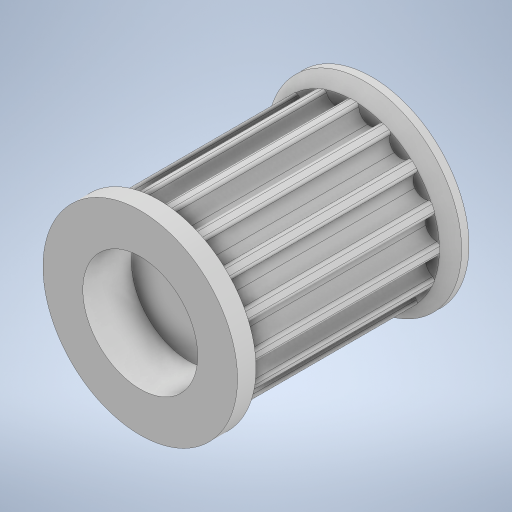
# Autodesk Inventor part: y_idler_teeth
Saved by Autodesk Inventor 2023 (Build 270158030, 158C)
## iProperties
Created: 2022-06-27
Part Number: y_idler_teeth
Material: 一般
Document SubType Name: Modeling
Designer: user
Density: 1 g/cm^3
Appearance: 預設
Author: user
## iProperties of the stored document y_idler_teeth_6mm_3D 列印.ipt
Created: 2022-06-29
Part Number: y_idler_teeth_6mm_3D 列印
Material: 一般
Document SubType Name: Modeling
Designer: user
Density: 1 g/cm^3
Appearance: 預設
Author: user
Autodesk Inventor part; units mm, degrees
ref_plane "YZ Plane" through (0, 0, 0) normal (1, 0, 0) x (0, 1, 0)
ref_plane "XZ Plane" through (0, 0, 0) normal (0, 1, 0) x (-1, 0, 0)
ref_plane "XY Plane" through (0, 0, 0) normal (0, 0, 1) x (1, 0, 0)
sketch "草圖1" plane through (0, 0, 0) normal (0, 0, 1) x (1, 0, 0)
  circle A0 centre (0, 0) radius 4
  arc A1 (0.305, 4.510097) -> (0.786957, 3.921823) centre (0.905, 4.510097) ccw
  arc A2 (-0.786957, 3.921823) -> (-0.305, 4.510097) centre (-0.905, 4.510097) ccw
  line L0 (0, -7) -> (0, 7)
  line L1 (-0.305, 4.510097) -> (0.305, 4.510097)
  line L2 (0.305, 4.510097) -> (0.305, 4.512097)
  line L3 (0.155, 4.662097) -> (-0.155, 4.662097)
  line L4 (-0.305, 4.512097) -> (-0.305, 4.510097)
  arc A3 (-0.155, 4.662097) -> (-0.305, 4.512097) centre (-0.155, 4.512097) ccw
  arc A4 (0.305, 4.512097) -> (0.155, 4.662097) centre (0.155, 4.512097) ccw
  circle A5 centre (0, 0) radius 3.1
  arc A6 (-2.22787, 3.322137) -> (-2.007723, 4.050068) centre (-2.56205, 3.820458) ccw
  line L5 (-1.640906, 4.366532) -> (-1.927309, 4.2479)
  arc A7 (-1.927309, 4.2479) -> (-2.008488, 4.051916) centre (-1.869906, 4.109318) ccw
  arc A8 (-1.444922, 4.285353) -> (-1.640906, 4.366532) centre (-1.583503, 4.22795) ccw
  arc A9 (-1.444156, 4.283505) -> (-0.773764, 3.924448) centre (-0.889828, 4.513115) ccw
  arc A10 (-3.32961, 2.216686) -> (-3.404788, 2.973453) centre (-3.829052, 2.549189) ccw
  line L6 (-3.186999, 3.406202) -> (-3.406202, 3.186999)
  arc A11 (-3.406202, 3.186999) -> (-3.406202, 2.974867) centre (-3.300136, 3.080933) ccw
  arc A12 (-2.974867, 3.406202) -> (-3.186999, 3.406202) centre (-3.080933, 3.300136) ccw
  arc A13 (-2.973453, 3.404788) -> (-2.216686, 3.32961) centre (-2.549189, 3.829052) ccw
  arc A14 (-3.924448, 0.773764) -> (-4.283505, 1.444156) centre (-4.513115, 0.889828) ccw
  line L7 (-4.2479, 1.927309) -> (-4.366532, 1.640906)
  arc A15 (-4.366532, 1.640906) -> (-4.285353, 1.444922) centre (-4.22795, 1.583503) ccw
  arc A16 (-4.051916, 2.008488) -> (-4.2479, 1.927309) centre (-4.109318, 1.869906) ccw
  arc A17 (-4.050068, 2.007723) -> (-3.322137, 2.22787) centre (-3.820458, 2.56205) ccw
  arc A18 (-3.921823, -0.786957) -> (-4.510097, -0.305) centre (-4.510097, -0.905) ccw
  line L8 (-4.662097, 0.155) -> (-4.662097, -0.155)
  arc A19 (-4.662097, -0.155) -> (-4.512097, -0.305) centre (-4.512097, -0.155) ccw
  arc A20 (-4.512097, 0.305) -> (-4.662097, 0.155) centre (-4.512097, 0.155) ccw
  arc A21 (-4.510097, 0.305) -> (-3.921823, 0.786957) centre (-4.510097, 0.905) ccw
  arc A22 (-3.322137, -2.22787) -> (-4.050068, -2.007723) centre (-3.820458, -2.56205) ccw
  line L9 (-4.366532, -1.640906) -> (-4.2479, -1.927309)
  arc A23 (-4.2479, -1.927309) -> (-4.051916, -2.008488) centre (-4.109318, -1.869906) ccw
  arc A24 (-4.285353, -1.444922) -> (-4.366532, -1.640906) centre (-4.22795, -1.583503) ccw
  arc A25 (-4.283505, -1.444156) -> (-3.924448, -0.773764) centre (-4.513115, -0.889828) ccw
  arc A26 (-2.216686, -3.32961) -> (-2.973453, -3.404788) centre (-2.549189, -3.829052) ccw
  line L10 (-3.406202, -3.186999) -> (-3.186999, -3.406202)
  arc A27 (-3.186999, -3.406202) -> (-2.974867, -3.406202) centre (-3.080933, -3.300136) ccw
  arc A28 (-3.406202, -2.974867) -> (-3.406202, -3.186999) centre (-3.300136, -3.080933) ccw
  arc A29 (-3.404788, -2.973453) -> (-3.32961, -2.216686) centre (-3.829052, -2.549189) ccw
  arc A30 (-0.773764, -3.924448) -> (-1.444156, -4.283505) centre (-0.889828, -4.513115) ccw
  line L11 (-1.927309, -4.2479) -> (-1.640906, -4.366532)
  arc A31 (-1.640906, -4.366532) -> (-1.444922, -4.285353) centre (-1.583503, -4.22795) ccw
  arc A32 (-2.008488, -4.051916) -> (-1.927309, -4.2479) centre (-1.869906, -4.109318) ccw
  arc A33 (-2.007723, -4.050068) -> (-2.22787, -3.322137) centre (-2.56205, -3.820458) ccw
  arc A34 (0.786957, -3.921823) -> (0.305, -4.510097) centre (0.905, -4.510097) ccw
  line L12 (-0.155, -4.662097) -> (0.155, -4.662097)
  arc A35 (0.155, -4.662097) -> (0.305, -4.512097) centre (0.155, -4.512097) ccw
  arc A36 (-0.305, -4.512097) -> (-0.155, -4.662097) centre (-0.155, -4.512097) ccw
  arc A37 (-0.305, -4.510097) -> (-0.786957, -3.921823) centre (-0.905, -4.510097) ccw
  arc A38 (2.22787, -3.322137) -> (2.007723, -4.050068) centre (2.56205, -3.820458) ccw
  line L13 (1.640906, -4.366532) -> (1.927309, -4.2479)
  arc A39 (1.927309, -4.2479) -> (2.008488, -4.051916) centre (1.869906, -4.109318) ccw
  arc A40 (1.444922, -4.285353) -> (1.640906, -4.366532) centre (1.583503, -4.22795) ccw
  arc A41 (1.444156, -4.283505) -> (0.773764, -3.924448) centre (0.889828, -4.513115) ccw
  arc A42 (3.32961, -2.216686) -> (3.404788, -2.973453) centre (3.829052, -2.549189) ccw
  line L14 (3.186999, -3.406202) -> (3.406202, -3.186999)
  arc A43 (3.406202, -3.186999) -> (3.406202, -2.974867) centre (3.300136, -3.080933) ccw
  arc A44 (2.974867, -3.406202) -> (3.186999, -3.406202) centre (3.080933, -3.300136) ccw
  arc A45 (2.973453, -3.404788) -> (2.216686, -3.32961) centre (2.549189, -3.829052) ccw
  arc A46 (3.924448, -0.773764) -> (4.283505, -1.444156) centre (4.513115, -0.889828) ccw
  line L15 (4.2479, -1.927309) -> (4.366532, -1.640906)
  arc A47 (4.366532, -1.640906) -> (4.285353, -1.444922) centre (4.22795, -1.583503) ccw
  arc A48 (4.051916, -2.008488) -> (4.2479, -1.927309) centre (4.109318, -1.869906) ccw
  arc A49 (4.050068, -2.007723) -> (3.322137, -2.22787) centre (3.820458, -2.56205) ccw
  arc A50 (3.921823, 0.786957) -> (4.510097, 0.305) centre (4.510097, 0.905) ccw
  line L16 (4.662097, -0.155) -> (4.662097, 0.155)
  arc A51 (4.662097, 0.155) -> (4.512097, 0.305) centre (4.512097, 0.155) ccw
  arc A52 (4.512097, -0.305) -> (4.662097, -0.155) centre (4.512097, -0.155) ccw
  arc A53 (4.510097, -0.305) -> (3.921823, -0.786957) centre (4.510097, -0.905) ccw
  arc A54 (3.322137, 2.22787) -> (4.050068, 2.007723) centre (3.820458, 2.56205) ccw
  line L17 (4.366532, 1.640906) -> (4.2479, 1.927309)
  arc A55 (4.2479, 1.927309) -> (4.051916, 2.008488) centre (4.109318, 1.869906) ccw
  arc A56 (4.285353, 1.444922) -> (4.366532, 1.640906) centre (4.22795, 1.583503) ccw
  arc A57 (4.283505, 1.444156) -> (3.924448, 0.773764) centre (4.513115, 0.889828) ccw
  arc A58 (2.216686, 3.32961) -> (2.973453, 3.404788) centre (2.549189, 3.829052) ccw
  line L18 (3.406202, 3.186999) -> (3.186999, 3.406202)
  arc A59 (3.186999, 3.406202) -> (2.974867, 3.406202) centre (3.080933, 3.300136) ccw
  arc A60 (3.406202, 2.974867) -> (3.406202, 3.186999) centre (3.300136, 3.080933) ccw
  arc A61 (3.404788, 2.973453) -> (3.32961, 2.216686) centre (3.829052, 2.549189) ccw
  arc A62 (0.773764, 3.924448) -> (1.444156, 4.283505) centre (0.889828, 4.513115) ccw
  line L19 (1.927309, 4.2479) -> (1.640906, 4.366532)
  arc A63 (1.640906, 4.366532) -> (1.444922, 4.285353) centre (1.583503, 4.22795) ccw
  arc A64 (2.008488, 4.051916) -> (1.927309, 4.2479) centre (1.869906, 4.109318) ccw
  arc A65 (2.007723, 4.050068) -> (2.22787, 3.322137) centre (2.56205, 3.820458) ccw
  circle A66 centre (0, 0) radius 5
  line L20 (-1.444925, 4.28536) -> (-1.444156, 4.283505)
  line L21 (-2.008488, 4.051916) -> (-2.007723, 4.050068)
  line L22 (-3.406202, 2.974867) -> (-3.404788, 2.973453)
  line L23 (-2.974873, 3.406208) -> (-2.973453, 3.404788)
  line L24 (-4.285353, 1.444922) -> (-4.283505, 1.444156)
  line L25 (-4.051923, 2.008491) -> (-4.050068, 2.007723)
  line L26 (-4.512097, -0.305) -> (-4.510097, -0.305)
  line L27 (-4.512105, 0.305) -> (-4.510097, 0.305)
  line L28 (-4.051916, -2.008488) -> (-4.050068, -2.007723)
  line L29 (-4.28536, -1.444925) -> (-4.283505, -1.444156)
  line L30 (-2.974867, -3.406202) -> (-2.973453, -3.404788)
  line L31 (-3.406208, -2.974873) -> (-3.404788, -2.973453)
  line L32 (-1.444922, -4.285353) -> (-1.444156, -4.283505)
  line L33 (-2.008491, -4.051923) -> (-2.007723, -4.050068)
  line L34 (0.305, -4.512097) -> (0.305, -4.510097)
  line L35 (-0.305, -4.512105) -> (-0.305, -4.510097)
  line L36 (2.008488, -4.051916) -> (2.007723, -4.050068)
  line L37 (1.444925, -4.28536) -> (1.444156, -4.283505)
  line L38 (3.406202, -2.974867) -> (3.404788, -2.973453)
  line L39 (2.974873, -3.406208) -> (2.973453, -3.404788)
  line L40 (4.285353, -1.444922) -> (4.283505, -1.444156)
  line L41 (4.051923, -2.008491) -> (4.050068, -2.007723)
  line L42 (4.512097, 0.305) -> (4.510097, 0.305)
  line L43 (4.512105, -0.305) -> (4.510097, -0.305)
  line L44 (4.051916, 2.008488) -> (4.050068, 2.007723)
  line L45 (4.28536, 1.444925) -> (4.283505, 1.444156)
  line L46 (2.974867, 3.406202) -> (2.973453, 3.404788)
  line L47 (3.406208, 2.974873) -> (3.404788, 2.973453)
  line L48 (1.444922, 4.285353) -> (1.444156, 4.283505)
  line L49 (2.008491, 4.051923) -> (2.007723, 4.050068)
  line L50 (-0.305, 4.512097) -> (-0.305, 4.510097)
  line L51 (0.305, 4.512105) -> (0.305, 4.510097)
  circle A67 centre (0, 0) radius 2
  point P0 (-0.78037, 3.923184)
  point P1 (-2.222305, 3.325914)
  point P2 (-3.404788, 2.973453)
  point P3 (-3.325914, 2.222305)
  point P4 (-3.923184, 0.78037)
  point P5 (-4.512097, 0.305)
  point P6 (-4.512097, -0.305)
  point P7 (-4.510097, -0.305)
  point P8 (-3.923184, -0.78037)
  point P9 (-4.283505, -1.444156)
  point P10 (-3.325914, -2.222305)
  point P11 (-2.222305, -3.325914)
  point P12 (-0.78037, -3.923184)
  point P13 (-0.305, -4.512097)
  point P14 (0.305, -4.512097)
  point P15 (0.78037, -3.923184)
  point P16 (2.222305, -3.325914)
  point P17 (3.325914, -2.222305)
  point P18 (4.283505, -1.444156)
  point P19 (3.923184, -0.78037)
  point P20 (4.512097, -0.305)
  point P21 (4.512097, 0.305)
  point P22 (3.923184, 0.78037)
  point P23 (4.283505, 1.444156)
  point P24 (4.051916, 2.008488)
  point P25 (3.325914, 2.222305)
  point P26 (2.973453, 3.404788)
  point P27 (2.222305, 3.325914)
  point P28 (1.444922, 4.285353)
  point P29 (0.78037, 3.923184)
  dimension "d0" = 8
  dimension "d1" = 1.2
  dimension "d2" = 0.61
  dimension "d3" = 0.15
  dimension "d4" = 0.152
  dimension "d5" = 6.2
  dimension "d8" = 360
  dimension "d10" = 10
  dimension "d13" = 360
  dimension "d20" = 4
  constraints: 130 point on circle, 102 end point, 68 centre point, 8 tangent, 4 coincident, 3 parallel, 1 equal radius, 1 horizontal, 1 perpendicular, 1 symmetric about line, 370 other
  measures "d0" diameter of A0
  measures "d1" diameter of A2
  measures "d2" distance of L1.start L1.end
  measures "d3" radius of A3
  measures "d4" distance between parallel lines of L1 L3
  measures "d5" diameter of A5
  measures "d10" diameter of A66
  measures "d20" diameter of A67
extrude "擠出1" add sketch "草圖1" along normal mid plane 10.5 contours A0 L0 A5 | A0 A50 A51 L16 A52 A53 | A0 A54 A55 L17 A56 A57 | A46 A47 L15 A48 A49 A0 | A0 A58 A59 L18 A60 A61 | A42 A43 L14 A44 A45 A0 | A0 A62 A63 L19 A64 A65 | A38 A39 L13 A40 A41 A0 | A0 L0 L1 A1 | A34 A35 L12 L0 A0 | L0 A5 A0 | A0 A2 L1 L0 | L1 L0 L3 A4 | L0 L12 A36 A37 A0 | L1 A3 L3 L0 | A0 A6 A7 L5 A8 A9 | A30 A31 L11 A32 A33 A0 | A0 A10 A11 L6 A12 A13 | A26 A27 L10 A28 A29 A0 | A0 A14 A15 L7 A16 A17 | A22 A23 L9 A24 A25 A0 | A0 A18 A19 L8 A20 A21
sketch "草圖2" plane through (0, 0, 5.25) normal (0, 0, 1) x (1, 0, 0)
  arc A0 (-1.444922, 4.285353) -> (-0.78037, 3.923184) centre (-0.889827, 4.513123) ccw
  arc A1 (-1.444922, 4.285353) -> (-1.640906, 4.366532) centre (-1.583503, 4.22795) ccw
  line L0 (-1.640906, 4.366532) -> (-1.927309, 4.2479)
  arc A2 (-1.927309, 4.2479) -> (-2.008488, 4.051916) centre (-1.869906, 4.109318) ccw
  arc A3 (-2.222305, 3.325914) -> (-2.008488, 4.051916) centre (-2.562057, 3.820462) ccw
  arc A4 (-2.974867, 3.406202) -> (-2.222305, 3.325914) centre (-2.54919, 3.829059) ccw
  arc A5 (-2.974867, 3.406202) -> (-3.186999, 3.406202) centre (-3.080933, 3.300136) ccw
  line L1 (-3.186999, 3.406202) -> (-3.406202, 3.186999)
  arc A6 (-3.406202, 3.186999) -> (-3.406202, 2.974867) centre (-3.300136, 3.080933) ccw
  arc A7 (-3.325914, 2.222305) -> (-3.406202, 2.974867) centre (-3.829059, 2.54919) ccw
  arc A8 (-4.051916, 2.008488) -> (-3.325914, 2.222305) centre (-3.820462, 2.562057) ccw
  arc A9 (-4.051916, 2.008488) -> (-4.2479, 1.927309) centre (-4.109318, 1.869906) ccw
  line L2 (-4.2479, 1.927309) -> (-4.366532, 1.640906)
  arc A10 (-4.366532, 1.640906) -> (-4.285353, 1.444922) centre (-4.22795, 1.583503) ccw
  arc A11 (-3.923184, 0.78037) -> (-4.285353, 1.444922) centre (-4.513123, 0.889827) ccw
  arc A12 (-4.512097, 0.305) -> (-3.923184, 0.78037) centre (-4.510104, 0.905004) ccw
  arc A13 (-4.512097, 0.305) -> (-4.662097, 0.155) centre (-4.512097, 0.155) ccw
  line L3 (-4.662097, 0.155) -> (-4.662097, -0.155)
  arc A14 (-4.662097, -0.155) -> (-4.512097, -0.305) centre (-4.512097, -0.155) ccw
  arc A15 (-3.923184, -0.78037) -> (-4.512097, -0.305) centre (-4.510104, -0.905004) ccw
  arc A16 (-4.285353, -1.444922) -> (-3.923184, -0.78037) centre (-4.513123, -0.889827) ccw
  arc A17 (-4.285353, -1.444922) -> (-4.366532, -1.640906) centre (-4.22795, -1.583503) ccw
  line L4 (-4.366532, -1.640906) -> (-4.2479, -1.927309)
  arc A18 (-4.2479, -1.927309) -> (-4.051916, -2.008488) centre (-4.109318, -1.869906) ccw
  arc A19 (-3.325914, -2.222305) -> (-4.051916, -2.008488) centre (-3.820462, -2.562057) ccw
  arc A20 (-3.406202, -2.974867) -> (-3.325914, -2.222305) centre (-3.829059, -2.54919) ccw
  arc A21 (-3.406202, -2.974867) -> (-3.406202, -3.186999) centre (-3.300136, -3.080933) ccw
  line L5 (-3.406202, -3.186999) -> (-3.186999, -3.406202)
  arc A22 (-3.186999, -3.406202) -> (-2.974867, -3.406202) centre (-3.080933, -3.300136) ccw
  arc A23 (-2.222305, -3.325914) -> (-2.974867, -3.406202) centre (-2.54919, -3.829059) ccw
  arc A24 (-2.008488, -4.051916) -> (-2.222305, -3.325914) centre (-2.562057, -3.820462) ccw
  arc A25 (-2.008488, -4.051916) -> (-1.927309, -4.2479) centre (-1.869906, -4.109318) ccw
  line L6 (-1.927309, -4.2479) -> (-1.640906, -4.366532)
  arc A26 (-1.640906, -4.366532) -> (-1.444922, -4.285353) centre (-1.583503, -4.22795) ccw
  arc A27 (-0.78037, -3.923184) -> (-1.444922, -4.285353) centre (-0.889827, -4.513123) ccw
  arc A28 (-0.305, -4.512097) -> (-0.78037, -3.923184) centre (-0.905004, -4.510104) ccw
  arc A29 (-0.305, -4.512097) -> (-0.155, -4.662097) centre (-0.155, -4.512097) ccw
  line L7 (-0.155, -4.662097) -> (0.155, -4.662097)
  arc A30 (0.155, -4.662097) -> (0.305, -4.512097) centre (0.155, -4.512097) ccw
  arc A31 (0.78037, -3.923184) -> (0.305, -4.512097) centre (0.905004, -4.510104) ccw
  arc A32 (1.444922, -4.285353) -> (0.78037, -3.923184) centre (0.889827, -4.513123) ccw
  arc A33 (1.444922, -4.285353) -> (1.640906, -4.366532) centre (1.583503, -4.22795) ccw
  line L8 (1.640906, -4.366532) -> (1.927309, -4.2479)
  arc A34 (1.927309, -4.2479) -> (2.008488, -4.051916) centre (1.869906, -4.109318) ccw
  arc A35 (2.222305, -3.325914) -> (2.008488, -4.051916) centre (2.562057, -3.820462) ccw
  arc A36 (2.974867, -3.406202) -> (2.222305, -3.325914) centre (2.54919, -3.829059) ccw
  arc A37 (2.974867, -3.406202) -> (3.186999, -3.406202) centre (3.080933, -3.300136) ccw
  line L9 (3.186999, -3.406202) -> (3.406202, -3.186999)
  arc A38 (3.406202, -3.186999) -> (3.406202, -2.974867) centre (3.300136, -3.080933) ccw
  arc A39 (3.325914, -2.222305) -> (3.406202, -2.974867) centre (3.829059, -2.54919) ccw
  arc A40 (4.051916, -2.008488) -> (3.325914, -2.222305) centre (3.820462, -2.562057) ccw
  arc A41 (4.051916, -2.008488) -> (4.2479, -1.927309) centre (4.109318, -1.869906) ccw
  line L10 (4.2479, -1.927309) -> (4.366532, -1.640906)
  arc A42 (4.366532, -1.640906) -> (4.285353, -1.444922) centre (4.22795, -1.583503) ccw
  arc A43 (3.923184, -0.78037) -> (4.285353, -1.444922) centre (4.513123, -0.889827) ccw
  arc A44 (4.512097, -0.305) -> (3.923184, -0.78037) centre (4.510104, -0.905004) ccw
  arc A45 (4.512097, -0.305) -> (4.662097, -0.155) centre (4.512097, -0.155) ccw
  line L11 (4.662097, -0.155) -> (4.662097, 0.155)
  arc A46 (4.662097, 0.155) -> (4.512097, 0.305) centre (4.512097, 0.155) ccw
  arc A47 (3.923184, 0.78037) -> (4.512097, 0.305) centre (4.510104, 0.905004) ccw
  arc A48 (4.285353, 1.444922) -> (3.923184, 0.78037) centre (4.513123, 0.889827) ccw
  arc A49 (4.285353, 1.444922) -> (4.366532, 1.640906) centre (4.22795, 1.583503) ccw
  line L12 (4.366532, 1.640906) -> (4.2479, 1.927309)
  arc A50 (4.2479, 1.927309) -> (4.051916, 2.008488) centre (4.109318, 1.869906) ccw
  arc A51 (3.325914, 2.222305) -> (4.051916, 2.008488) centre (3.820462, 2.562057) ccw
  arc A52 (3.406202, 2.974867) -> (3.325914, 2.222305) centre (3.829059, 2.54919) ccw
  arc A53 (3.406202, 2.974867) -> (3.406202, 3.186999) centre (3.300136, 3.080933) ccw
  line L13 (3.406202, 3.186999) -> (3.186999, 3.406202)
  arc A54 (3.186999, 3.406202) -> (2.974867, 3.406202) centre (3.080933, 3.300136) ccw
  arc A55 (2.222305, 3.325914) -> (2.974867, 3.406202) centre (2.54919, 3.829059) ccw
  arc A56 (2.008488, 4.051916) -> (2.222305, 3.325914) centre (2.562057, 3.820462) ccw
  arc A57 (2.008488, 4.051916) -> (1.927309, 4.2479) centre (1.869906, 4.109318) ccw
  line L14 (1.927309, 4.2479) -> (1.640906, 4.366532)
  arc A58 (1.640906, 4.366532) -> (1.444922, 4.285353) centre (1.583503, 4.22795) ccw
  arc A59 (0.78037, 3.923184) -> (1.444922, 4.285353) centre (0.889827, 4.513123) ccw
  arc A60 (0.305, 4.512097) -> (0.78037, 3.923184) centre (0.905004, 4.510104) ccw
  arc A61 (0.305, 4.512097) -> (0.155, 4.662097) centre (0.155, 4.512097) ccw
  line L15 (0.155, 4.662097) -> (-0.155, 4.662097)
  arc A62 (-0.155, 4.662097) -> (-0.305, 4.512097) centre (-0.155, 4.512097) ccw
  arc A63 (-0.78037, 3.923184) -> (-0.305, 4.512097) centre (-0.905004, 4.510104) ccw
  circle A64 centre (0, 0) radius 3.1
  circle A65 centre (0, 0) radius 5.25
  dimension "d17" = 10.5
  constraints: 1 centre point, 1 coincident
  measures "d17" diameter of A65
extrude "擠出2" add sketch "草圖2" along normal blind 1 contours A0 A63 A62 L15 A61 A60 A59 A58 L14 A57 A56 A55 A54 L13 A53 A52 A51 A50 L12 A49 A48 A47 A46 L11 A45 A44 A43 A42 L10 A41 A40 A39 A38 L9 A37 A36 A35 A34 L8 A33 A32 A31 A30 L7 A29 A28 A27 A26 L6 A25 A24 A23 A22 L5 A21 A20 A19 A18 L4 A17 A16 A15 A14 L3 A13 A12 A11 A10 L2 A9 A8 A7 A6 L1 A5 A4 A3 A2 L0 A1 | A65
mirror "鏡射1" about plane through (0, 0, 0) normal (0, 0, 1) of "擠出2"
extrude "擠出3" add sketch "草圖1" along normal mid plane 7.25 contours A5 L0 A67 | L0 A67 A5
sketch "草圖3" plane through (0, 0, 3.625) normal (0, 0, 1) x (1, 0, 0)
  circle A0 centre (0, 0) radius 2
  circle A1 centre (0, 0) radius 3.1
  arc A2 (-0.78037, 3.923184) -> (-0.305, 4.512097) centre (-0.905004, 4.510104) ccw
  arc A3 (-0.155, 4.662097) -> (-0.305, 4.512097) centre (-0.155, 4.512097) ccw
  line L0 (-0.155, 4.662097) -> (0.155, 4.662097)
  arc A4 (0.305, 4.512097) -> (0.155, 4.662097) centre (0.155, 4.512097) ccw
  arc A5 (0.305, 4.512097) -> (0.78037, 3.923184) centre (0.905004, 4.510104) ccw
  arc A6 (0.78037, 3.923184) -> (1.444922, 4.285353) centre (0.889827, 4.513123) ccw
  arc A7 (1.640906, 4.366532) -> (1.444922, 4.285353) centre (1.583503, 4.22795) ccw
  line L1 (1.640906, 4.366532) -> (1.927309, 4.2479)
  arc A8 (2.008488, 4.051916) -> (1.927309, 4.2479) centre (1.869906, 4.109318) ccw
  arc A9 (2.008488, 4.051916) -> (2.222305, 3.325914) centre (2.562057, 3.820462) ccw
  arc A10 (2.222305, 3.325914) -> (2.974867, 3.406202) centre (2.54919, 3.829059) ccw
  arc A11 (3.186999, 3.406202) -> (2.974867, 3.406202) centre (3.080933, 3.300136) ccw
  line L2 (3.186999, 3.406202) -> (3.406202, 3.186999)
  arc A12 (3.406202, 2.974867) -> (3.406202, 3.186999) centre (3.300136, 3.080933) ccw
  arc A13 (3.406202, 2.974867) -> (3.325914, 2.222305) centre (3.829059, 2.54919) ccw
  arc A14 (3.325914, 2.222305) -> (4.051916, 2.008488) centre (3.820462, 2.562057) ccw
  arc A15 (4.2479, 1.927309) -> (4.051916, 2.008488) centre (4.109318, 1.869906) ccw
  line L3 (4.2479, 1.927309) -> (4.366532, 1.640906)
  arc A16 (4.285353, 1.444922) -> (4.366532, 1.640906) centre (4.22795, 1.583503) ccw
  arc A17 (4.285353, 1.444922) -> (3.923184, 0.78037) centre (4.513123, 0.889827) ccw
  arc A18 (3.923184, 0.78037) -> (4.512097, 0.305) centre (4.510104, 0.905004) ccw
  arc A19 (4.662097, 0.155) -> (4.512097, 0.305) centre (4.512097, 0.155) ccw
  line L4 (4.662097, 0.155) -> (4.662097, -0.155)
  arc A20 (4.512097, -0.305) -> (4.662097, -0.155) centre (4.512097, -0.155) ccw
  arc A21 (4.512097, -0.305) -> (3.923184, -0.78037) centre (4.510104, -0.905004) ccw
  arc A22 (3.923184, -0.78037) -> (4.285353, -1.444922) centre (4.513123, -0.889827) ccw
  arc A23 (4.366532, -1.640906) -> (4.285353, -1.444922) centre (4.22795, -1.583503) ccw
  line L5 (4.366532, -1.640906) -> (4.2479, -1.927309)
  arc A24 (4.051916, -2.008488) -> (4.2479, -1.927309) centre (4.109318, -1.869906) ccw
  arc A25 (4.051916, -2.008488) -> (3.325914, -2.222305) centre (3.820462, -2.562057) ccw
  arc A26 (3.325914, -2.222305) -> (3.406202, -2.974867) centre (3.829059, -2.54919) ccw
  arc A27 (3.406202, -3.186999) -> (3.406202, -2.974867) centre (3.300136, -3.080933) ccw
  line L6 (3.406202, -3.186999) -> (3.186999, -3.406202)
  arc A28 (2.974867, -3.406202) -> (3.186999, -3.406202) centre (3.080933, -3.300136) ccw
  arc A29 (2.974867, -3.406202) -> (2.222305, -3.325914) centre (2.54919, -3.829059) ccw
  arc A30 (2.222305, -3.325914) -> (2.008488, -4.051916) centre (2.562057, -3.820462) ccw
  arc A31 (1.927309, -4.2479) -> (2.008488, -4.051916) centre (1.869906, -4.109318) ccw
  line L7 (1.927309, -4.2479) -> (1.640906, -4.366532)
  arc A32 (1.444922, -4.285353) -> (1.640906, -4.366532) centre (1.583503, -4.22795) ccw
  arc A33 (1.444922, -4.285353) -> (0.78037, -3.923184) centre (0.889827, -4.513123) ccw
  arc A34 (0.78037, -3.923184) -> (0.305, -4.512097) centre (0.905004, -4.510104) ccw
  arc A35 (0.155, -4.662097) -> (0.305, -4.512097) centre (0.155, -4.512097) ccw
  line L8 (0.155, -4.662097) -> (-0.155, -4.662097)
  arc A36 (-0.305, -4.512097) -> (-0.155, -4.662097) centre (-0.155, -4.512097) ccw
  arc A37 (-0.305, -4.512097) -> (-0.78037, -3.923184) centre (-0.905004, -4.510104) ccw
  arc A38 (-0.78037, -3.923184) -> (-1.444922, -4.285353) centre (-0.889827, -4.513123) ccw
  arc A39 (-1.640906, -4.366532) -> (-1.444922, -4.285353) centre (-1.583503, -4.22795) ccw
  line L9 (-1.640906, -4.366532) -> (-1.927309, -4.2479)
  arc A40 (-2.008488, -4.051916) -> (-1.927309, -4.2479) centre (-1.869906, -4.109318) ccw
  arc A41 (-2.008488, -4.051916) -> (-2.222305, -3.325914) centre (-2.562057, -3.820462) ccw
  arc A42 (-2.222305, -3.325914) -> (-2.974867, -3.406202) centre (-2.54919, -3.829059) ccw
  arc A43 (-3.186999, -3.406202) -> (-2.974867, -3.406202) centre (-3.080933, -3.300136) ccw
  line L10 (-3.186999, -3.406202) -> (-3.406202, -3.186999)
  arc A44 (-3.406202, -2.974867) -> (-3.406202, -3.186999) centre (-3.300136, -3.080933) ccw
  arc A45 (-3.406202, -2.974867) -> (-3.325914, -2.222305) centre (-3.829059, -2.54919) ccw
  arc A46 (-3.325914, -2.222305) -> (-4.051916, -2.008488) centre (-3.820462, -2.562057) ccw
  arc A47 (-4.2479, -1.927309) -> (-4.051916, -2.008488) centre (-4.109318, -1.869906) ccw
  line L11 (-4.2479, -1.927309) -> (-4.366532, -1.640906)
  arc A48 (-4.285353, -1.444922) -> (-4.366532, -1.640906) centre (-4.22795, -1.583503) ccw
  arc A49 (-4.285353, -1.444922) -> (-3.923184, -0.78037) centre (-4.513123, -0.889827) ccw
  arc A50 (-3.923184, -0.78037) -> (-4.512097, -0.305) centre (-4.510104, -0.905004) ccw
  arc A51 (-4.662097, -0.155) -> (-4.512097, -0.305) centre (-4.512097, -0.155) ccw
  line L12 (-4.662097, -0.155) -> (-4.662097, 0.155)
  arc A52 (-4.512097, 0.305) -> (-4.662097, 0.155) centre (-4.512097, 0.155) ccw
  arc A53 (-4.512097, 0.305) -> (-3.923184, 0.78037) centre (-4.510104, 0.905004) ccw
  arc A54 (-3.923184, 0.78037) -> (-4.285353, 1.444922) centre (-4.513123, 0.889827) ccw
  arc A55 (-4.366532, 1.640906) -> (-4.285353, 1.444922) centre (-4.22795, 1.583503) ccw
  line L13 (-4.366532, 1.640906) -> (-4.2479, 1.927309)
  arc A56 (-4.051916, 2.008488) -> (-4.2479, 1.927309) centre (-4.109318, 1.869906) ccw
  arc A57 (-4.051916, 2.008488) -> (-3.325914, 2.222305) centre (-3.820462, 2.562057) ccw
  arc A58 (-3.325914, 2.222305) -> (-3.406202, 2.974867) centre (-3.829059, 2.54919) ccw
  arc A59 (-3.406202, 3.186999) -> (-3.406202, 2.974867) centre (-3.300136, 3.080933) ccw
  line L14 (-3.406202, 3.186999) -> (-3.186999, 3.406202)
  arc A60 (-2.974867, 3.406202) -> (-3.186999, 3.406202) centre (-3.080933, 3.300136) ccw
  arc A61 (-2.974867, 3.406202) -> (-2.222305, 3.325914) centre (-2.54919, 3.829059) ccw
  arc A62 (-2.222305, 3.325914) -> (-2.008488, 4.051916) centre (-2.562057, 3.820462) ccw
  arc A63 (-1.927309, 4.2479) -> (-2.008488, 4.051916) centre (-1.869906, 4.109318) ccw
  line L15 (-1.927309, 4.2479) -> (-1.640906, 4.366532)
  arc A64 (-1.444922, 4.285353) -> (-1.640906, 4.366532) centre (-1.583503, 4.22795) ccw
  arc A65 (-1.444922, 4.285353) -> (-0.78037, 3.923184) centre (-0.889827, 4.513123) ccw
extrude "擠出4" add sketch "草圖3" against normal blind 0.2 contours A0
chamfer "倒角1" distance 0.6 angle 45 1 edges at (-5.25, 0, -5.25)
